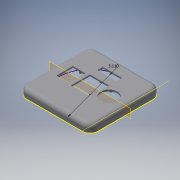
# Autodesk Inventor part: Body
Saved by Autodesk Inventor 2017 (Build 210142000, 142)
## iProperties
Created: 2017-02-21
Part Number: Body
Material: Generic
Document SubType Name: Modeling
Designer: prosp
Density: 1 g/cm^3
Appearance: Default
Author: prosp
Autodesk Inventor part; units mm, degrees
ref_plane "YZ Plane" through (0, 0, 0) normal (1, 0, 0) x (0, 1, 0)
ref_plane "XZ Plane" through (0, 0, 0) normal (0, 1, 0) x (-1, 0, 0)
sketch "Sketch1" plane through (0, 0, 0) normal (0, 1, 0) x (-1, 0, 0)
  line L0 (45, 35) -> (45, -35)
  line L1 (35, -45) -> (-35, -45)
  line L2 (-45, -35) -> (-45, 35)
  line L3 (-35, 45) -> (35, 45)
  line L4 (45, 45) -> (-45, -45) construction
  line L5 (45, -45) -> (-45, 45) construction
  arc A0 (35, -45) -> (45, -35) centre (35, -35) ccw
  arc A1 (-45, -35) -> (-35, -45) centre (-35, -35) ccw
  arc A2 (-35, 45) -> (-45, 35) centre (-35, 35) ccw
  arc A3 (45, 35) -> (35, 45) centre (35, 35) ccw
  point P0 (0, 0)
  dimension "d0" = 90
  dimension "d1" = 90
  dimension "d10" = 10
  constraints: 12 end point, 8 point on circle, 8 point on line, 8 tangent, 4 centre point, 3 equal radius, 2 midpoint, 2 parallel, 1 perpendicular, 1 vertical
  measures "d0" distance of L4.start L5.start
  measures "d1" distance of L5.start L4.end
  measures "d10" radius of A0
extrude "Extrusion1" add sketch "Sketch1" along normal blind 10
shell "Shell2" thickness 2 removed faces 1 at (-11.6667, 0, -15)
fillet "Fillet1" radius 5 1 edges at (-45, 10, 0)
sketch "Sketch2" plane through (0, 10, 0) normal (0, 1, 0) x (1, 0, 0)
  circle A0 centre (24.0106, 0) radius 10 projected
  line L0 (-11.5, 11.5) -> (11.5, 11.5) projected
  line L1 (-11.5, -11.5) -> (-11.5, 11.5) projected
  line L2 (11.5, -11.5) -> (-11.5, -11.5) projected
  line L3 (11.5, 11.5) -> (11.5, -11.5) projected
  line L4 (-31.5, -10) -> (-16.5, -10) projected
  line L5 (-16.5, -10) -> (-16.5, 10) projected
  line L6 (-16.5, 10) -> (-31.5, 10) projected
  line L7 (-31.5, 10) -> (-31.5, -10) projected
  line L8 (-11.5, 22) -> (11.5, 22) projected
  line L9 (11.5, 22) -> (11.5, 28) projected
  line L10 (11.5, 28) -> (-11.5, 28) projected
  line L11 (-11.5, 28) -> (-11.5, 22) projected
  line L12 (12, 21.5) -> (-12, 21.5)
  line L13 (-12, 21.5) -> (-12, 28.5)
  line L14 (-12, 28.5) -> (12, 28.5)
  line L15 (12, 28.5) -> (12, 21.5)
  circle A1 centre (24.0106, 0) radius 10.5
  line L16 (12, 12) -> (-12, 12)
  line L17 (-12, 12) -> (-12, -12)
  line L18 (-12, -12) -> (12, -12)
  line L19 (12, -12) -> (12, 12)
  line L20 (-16, 10.5) -> (-16, -10.5)
  line L21 (-16, -10.5) -> (-32, -10.5)
  line L22 (-32, -10.5) -> (-32, 10.5)
  line L23 (-32, 10.5) -> (-16, 10.5)
  point P0 (0, 0)
  dimension "d13" = 0.5
  dimension "d14" = 0.5
  dimension "d15" = 0.5
  dimension "d16" = 0.5
  constraints: 24 end point, 1 centre point, 9 other
  measures "d13" distance between parallel lines of L15 L9
  measures "d14" distance between parallel lines of L23 L6
  measures "d15" distance between parallel lines of L16 L0
  measures "d16" radial gap between concentric circles of A0 A1
extrude "Extrusion2" cut sketch "Sketch2" along normal through all both and the other way through all contours A0 | L0 L3 L2 L1 | L7 L6 L5 L4 | L11 L10 L9 L8 | L12 L13 L14 L15 | A1 | L19 L18 L17 L16 | L20 L21 L22 L23
sketch "Sketch3" plane through (-35, 8, -43) normal (0, -1, 0) x (1, 0, 0)
  circle A0 centre (35, 28.5) radius 1 projected
  circle A1 centre (35, 57.5) radius 1 projected
  circle A2 centre (51.5106, 33) radius 1.5 projected
  circle A3 centre (66.5106, 33) radius 1.5 projected
  circle A4 centre (51.5106, 60.4954) radius 1.5 projected
  circle A5 centre (66.5106, 60.5) radius 1.5 projected
  circle A6 centre (11, 31) radius 1.5 projected
  arc A7 (37, 28.5) -> (33, 28.5) centre (35, 28.5) ccw
  circle A8 centre (35, 57.5) radius 2
  circle A9 centre (51.5106, 33) radius 2
  circle A10 centre (51.5106, 60.4954) radius 2
  circle A11 centre (66.5106, 60.5) radius 2
  circle A12 centre (66.5106, 33) radius 2
  circle A13 centre (11, 31) radius 1.35
  arc A14 (33, 26) -> (37, 26) centre (35, 26) ccw
  line L0 (53.5, 23) -> (15.5, 23) projected
  line L1 (33, 28.5) -> (33, 26)
  line L2 (37, 28.5) -> (37, 26)
  point P0 (35, 43)
  dimension "d19" = 4
  dimension "d20" = 4
  dimension "d21" = 4
  dimension "d22" = 2.7
  dimension "d32" = 3
  constraints: 8 centre point, 7 coincident, 4 end point, 4 equal radius, 4 point on circle, 4 tangent, 1 vertical alignment
  measures "d19" diameter of A7
  measures "d20" diameter of A8
  measures "d21" diameter of A9
  measures "d22" diameter of A13
  measures "d32" distance from line of L0 A14.centre
extrude "Extrusion3" add sketch "Sketch3" along normal blind 1.4986 contours A0 | A1 | L2 A14 L1 A7 | A8
sketch "Sketch4" plane through (-35, 8, -43) normal (0, -1, 0) x (1, 0, 0)
  circle A0 centre (51.5106, 60.4954) radius 2 projected
  circle A1 centre (66.5106, 60.5) radius 2 projected
  circle A2 centre (66.5106, 33) radius 2 projected
  circle A3 centre (51.5106, 33) radius 2 projected
  point P0 (35, 43)
extrude "Extrusion4" add sketch "Sketch4" along normal blind 0.9906
sketch "Sketch5" plane through (-35, 8, -43) normal (0, -1, 0) x (1, 0, 0)
  circle A0 centre (11, 31) radius 1.35 projected
  point P0 (35, 43)
extrude "Extrusion5" add sketch "Sketch5" along normal blind 2.4892
sketch "Sketch6" plane through (-35, 8, -43) normal (0, -1, 0) x (1, 0, 0)
  circle A0 centre (35, 8) radius 2
  circle A1 centre (35, 28.5) radius 2 projected
  line L0 (15.5, 11) -> (53.5, 11) projected
  point P0 (35, 43)
  dimension "d29" = 3
  constraints: 1 centre point, 1 equal radius, 1 vertical alignment
  measures "d29" distance from line of L0 A0.centre
extrude "Extrusion6" add sketch "Sketch6" along normal blind 1.4986 contours A0
sketch "Sketch7" plane through (31.5106, 7.0094, 17.5) normal (0, -1, 0) x (1, 0, 0)
  circle A0 centre (0, 0) radius 2 projected
  circle A1 centre (-15, -0.0046) radius 2 projected
  circle A2 centre (-31.5106, -3) radius 2 projected
  circle A3 centre (-31.5106, -52.5) radius 2 projected
  circle A4 centre (-55.5106, -29.5) radius 1.35 projected
  line L0 (3.4894, -60.5) -> (-66.5106, -60.5) projected
  arc A5 (3.4894, -60.5) -> (11.4894, -52.5) centre (3.4894, -52.5) ccw projected
  line L1 (11.4894, 17.5) -> (11.4894, -52.5) projected
  arc A6 (11.4894, 17.5) -> (3.4894, 25.5) centre (3.4894, 17.5) ccw projected
  line L2 (-66.5106, 25.5) -> (3.4894, 25.5) projected
  arc A7 (-66.5106, 25.5) -> (-74.5106, 17.5) centre (-66.5106, 17.5) ccw projected
  line L3 (-74.5106, -52.5) -> (-74.5106, 17.5) projected
  arc A8 (-74.5106, -52.5) -> (-66.5106, -60.5) centre (-66.5106, -52.5) ccw projected
  line L4 (-19.5106, -5.5) -> (-19.5106, -29.5) projected
  line L5 (-19.5106, -29.5) -> (-43.5106, -29.5) projected
  line L6 (-43.5106, -29.5) -> (-43.5106, -5.5) projected
  line L7 (-43.5106, -5.5) -> (-19.5106, -5.5) projected
  line L8 (-63.5106, -7) -> (-47.5106, -7) projected
  line L9 (-47.5106, -7) -> (-47.5106, -28) projected
  line L10 (-47.5106, -28) -> (-63.5106, -28) projected
  line L11 (-63.5106, -28) -> (-63.5106, -7) projected
  line L12 (-43.5106, -46) -> (-43.5106, -39) projected
  line L13 (-43.5106, -39) -> (-19.5106, -39) projected
  line L14 (-19.5106, -39) -> (-19.5106, -46) projected
  line L15 (-19.5106, -46) -> (-43.5106, -46) projected
  arc A9 (-1.2, -25.9) -> (-13.8, -25.9) centre (-7.5, -17.5) ccw projected
  circle A10 centre (0, -27.5) radius 2 projected
  arc A11 (-13.8, -25.9) -> (-1.2, -25.9) centre (-7.5, -17.5) ccw projected
  circle A12 centre (-15, -27.5) radius 2 projected
  circle A13 centre (-31.5106, -3) radius 2 projected
  arc A14 (-29.5106, -32) -> (-33.5106, -32) centre (-31.5106, -32) ccw projected
  line L16 (-29.5106, -32) -> (-29.5106, -34.5) projected
  arc A15 (-33.5106, -34.5) -> (-29.5106, -34.5) centre (-31.5106, -34.5) ccw projected
  line L17 (-33.5106, -34.5) -> (-33.5106, -32) projected
  circle A16 centre (0, 0) radius 2 projected
  circle A17 centre (-15, -0.0046) radius 2 projected
  circle A18 centre (0, 0) radius 0.75
  circle A19 centre (-15, -0.0046) radius 2 projected
  circle A20 centre (-15, -0.0046) radius 0.75
  circle A21 centre (-31.5106, -3) radius 2 projected
  circle A22 centre (-31.5106, -3) radius 0.75
  circle A23 centre (-15, -27.5) radius 2 projected
  circle A24 centre (-15, -27.5) radius 0.75
  arc A25 (-29.5106, -32) -> (-33.5106, -32) centre (-31.5106, -32) ccw projected
  circle A26 centre (-31.5106, -32) radius 0.75
  circle A27 centre (0, -27.5) radius 0.75
  circle A28 centre (-31.5106, -35) radius 0.75
  circle A29 centre (-55.5106, -29.5) radius 0.5
  circle A30 centre (-31.5106, -52.5) radius 0.75
  point P0 (-31.5106, -17.5)
  dimension "d33" = 0.5
  dimension "d34" = 1.5
  dimension "d35" = 1
  constraints: 9 centre point, 8 coincident, 7 equal radius, 1 vertical alignment, 3 other
  measures "d33" distance of A15.centre A28.centre
  measures "d34" diameter of A26
  measures "d35" diameter of A29
extrude "Extrusion7" cut sketch "Sketch7" along normal mid plane 4 contours A18 | A20 | A22 | A24 | A26 | A27 | A28 | A29 | A30
sketch "Sketch8" plane through (0, 0, 0) normal (0, -1, 0) x (1, 0, 0)
  arc A0 (35, -43) -> (43, -35) centre (35, -35) ccw projected
  line L0 (35, -43) -> (-35, -43) projected
  arc A1 (-43, -35) -> (-35, -43) centre (-35, -35) ccw projected
  line L1 (-43, -35) -> (-43, 35) projected
  arc A2 (-35, 43) -> (-43, 35) centre (-35, 35) ccw projected
  line L2 (-35, 43) -> (35, 43) projected
  arc A3 (43, 35) -> (35, 43) centre (35, 35) ccw projected
  line L3 (43, 35) -> (43, -35) projected
  line L4 (-35, -45) -> (35, -45) projected
  arc A4 (35, -45) -> (45, -35) centre (35, -35) ccw projected
  line L5 (45, -35) -> (45, 35) projected
  arc A5 (45, 35) -> (35, 45) centre (35, 35) ccw projected
  line L6 (35, 45) -> (-35, 45) projected
  arc A6 (-35, 45) -> (-45, 35) centre (-35, 35) ccw projected
  line L7 (-45, 35) -> (-45, -35) projected
  arc A7 (-45, -35) -> (-35, -45) centre (-35, -35) ccw projected
  circle A8 centre (0, 0) radius 39.5
  dimension "d38" = 79
  constraints: 1 centre point, 1 coincident
  measures "d38" diameter of A8
equation "\"d13\" = d14"
equation "\"d15\" = d14"
equation "\"d16\" = d14"
body "Solid1"
